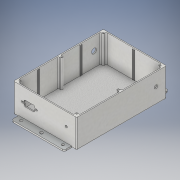
# Autodesk Inventor part: Main Enclosure Base
Saved by Autodesk Inventor 2019 (Build 230136000, 136)
## iProperties
Created: 2020-02-20
Part Number: Main Enclosure Base
Material: Generic
Document SubType Name: Modeling
Designer: gfb14170
Density: 1 g/cm^3
Appearance: Paint
Author: gfb14170
Autodesk Inventor part; units mm, degrees
ref_plane "YZ Plane" through (0, 0, 0) normal (1, 0, 0) x (0, 1, 0)
ref_plane "XZ Plane" through (0, 0, 0) normal (0, 1, 0) x (-1, 0, 0)
ref_plane "XY Plane" through (0, 0, 0) normal (0, 0, 1) x (1, 0, 0)
sketch "Sketch1" plane through (0, 0, 0) normal (0, 1, 0) x (-1, 0, 0)
  line L0 (60.4, 85.9) -> (-60.4, 85.9)
  line L1 (-60.4, 85.9) -> (-60.4, -85.9)
  line L2 (-60.4, -85.9) -> (60.4, -85.9)
  line L3 (60.4, -85.9) -> (60.4, 85.9)
  point P0 (0, 0)
  dimension "d0" = 85.9
  dimension "d1" = 85.9
  dimension "d2" = 60.4
  dimension "d3" = 60.4
  constraints: 8 end point, 2 parallel, 1 horizontal, 1 perpendicular
  measures "d0" distance from line of point (0, 0) L2
  measures "d1" distance from line of L0 point (0, 0)
  measures "d2" distance from line of point (0, 0) L3
  measures "d3" distance from line of L1 point (0, 0)
extrude "Extrusion1" add sketch "Sketch1" along normal blind 55.05
fillet "Fillet1" radius 2 6 edges at (60.4, 27.525, 85.9) (-60.4, 27.525, 85.9) (60.4, 27.525, -85.9) (-60.4, 27.525, -85.9) (60.4, 0, 0) (-60.4, 0, 0)
sketch "Sketch2" plane through (0, 55.05, 0) normal (0, 1, 0) x (1, 0, 0)
  line L0 (-58.4, -83.9) -> (58.4, -83.9)
  line L1 (58.4, -83.9) -> (58.4, 83.9)
  line L2 (58.4, 83.9) -> (-58.4, 83.9)
  line L3 (-58.4, 83.9) -> (-58.4, -83.9)
  line L4 (-60.4, 83.9) -> (-60.4, -83.9) projected
  line L5 (-58.4, -85.9) -> (58.4, -85.9) projected
  line L6 (60.4, -83.9) -> (60.4, 83.9) projected
  line L7 (58.4, 85.9) -> (-58.4, 85.9) projected
  point P0 (0, 0)
  dimension "d7" = 2
  dimension "d8" = 2
  dimension "d9" = 2
  dimension "d10" = 2
  constraints: 8 end point, 2 parallel, 1 horizontal, 1 perpendicular
  measures "d7" distance between parallel lines of L4 L3
  measures "d8" distance between parallel lines of L5 L0
  measures "d9" distance between parallel lines of L6 L1
  measures "d10" distance between parallel lines of L7 L2
extrude "Extrusion2" cut sketch "Sketch2" against normal blind 53.05
sketch "Sketch3" plane through (0, 0, 0) normal (0, -1, 0) x (1, 0, 0)
  line L0 (-58.4, -85.9) -> (-58.4, 85.9) projected
  line L1 (58.4, -85.9) -> (-58.4, -85.9) projected
  line L2 (58.4, 85.9) -> (58.4, -85.9) projected
  line L3 (-58.4, 85.9) -> (58.4, 85.9) projected
  line L4 (-58.4, 85.9) -> (58.4, 85.9) projected
  line L5 (50.4, 85.9) -> (50.4, 99.9)
  line L6 (50.4, 99.9) -> (-50.4, 99.9)
  line L7 (-50.4, 99.9) -> (-50.4, 85.9)
  line L8 (-60.4, 83.9) -> (-60.4, -83.9) projected
  line L9 (60.4, -83.9) -> (60.4, 83.9) projected
  line L10 (-134.6994, 0) -> (135.5184, 0) construction
  line L11 (50.4, -85.9) -> (50.4, -99.9)
  line L12 (50.4, -99.9) -> (-50.4, -99.9)
  line L13 (-50.4, -99.9) -> (-50.4, -85.9)
  line L14 (50.4, 85.9) -> (-50.4, 85.9)
  line L15 (-50.4, -85.9) -> (50.4, -85.9)
  point P0 (0, 0)
  dimension "d13" = 10
  dimension "d14" = 10
  dimension "d15" = 14
  dimension "d16" = 0
  constraints: 18 end point, 4 symmetric about line, 2 parallel, 1 collinear, 1 horizontal, 1 point on line
  measures "d13" distance between parallel lines of L8 L7
  measures "d14" distance between parallel lines of L5 L9
  measures "d15" distance between parallel lines of L3 L6
  measures "d16" distance from line of point (0, 0) L10
extrude "Extrusion3" add sketch "Sketch3" against normal blind 3 contours L1 L11 L12 L13 | L7 L6 L5 L3
fillet "Fillet2" radius 4 4 edges at (-50.4, 1.5, -99.9) (50.4, 1.5, -99.9) (50.4, 1.5, 99.9) (-50.4, 1.5, 99.9)
fillet "Fillet3" radius 2 8 edges at (-59.8142, 0.5858, 85.3142) (-54.4, 0, 85.9) (59.8142, 0.5858, 85.3142) (54.4, 0, 85.9) (59.8142, 0.5858, -85.3142) (54.4, 0, -85.9) (-59.8142, 0.5858, -85.3142) (-54.4, 0, -85.9)
sketch "Sketch4" plane through (0, 2, 0) normal (0, 1, 0) x (1, 0, 0)
  circle A0 centre (-54.9, 80.4) radius 1.25
  line L0 (58.4, 85.9) -> (-58.4, 85.9) projected
  line L1 (-60.4, 83.9) -> (-60.4, -83.9) projected
  circle A1 centre (54.1, 80.4) radius 1.25
  circle A2 centre (-54.9, -79.6) radius 1.25
  circle A3 centre (54.1, -79.6) radius 1.25
  circle A4 centre (-54.9, 80.4) radius 2.25
  circle A5 centre (-54.9, -79.6) radius 2.25
  circle A6 centre (54.1, 80.4) radius 2.25
  circle A7 centre (54.1, -79.6) radius 2.25
  line L2 (-58.4, 83.9) -> (-60.4, 83.9) projected
  line L3 (-58.4, 83.9) -> (-58.4, 75.9)
  line L4 (-58.4, 83.9) -> (-58.4, -83.9) projected
  line L5 (-58.4, 85.9) -> (-58.4, 83.9) projected
  line L6 (-58.4, 83.9) -> (-50.4, 83.9)
  line L7 (-58.4, 83.9) -> (58.4, 83.9) projected
  arc A8 (-55.4407, 78.2159) -> (-58.4, 75.9) centre (-56.0141, 75.9) ccw
  arc A9 (-50.4, 83.9) -> (-52.7159, 80.9407) centre (-50.4, 81.5141) ccw
  line L8 (58.4, 83.9) -> (58.4, -83.9) projected
  line L9 (58.4, 83.9) -> (50.4, 83.9)
  line L10 (58.4, 83.9) -> (58.4, 75.9)
  line L11 (58.4, -83.9) -> (58.4, 83.9) projected
  arc A10 (52.0522, 81.3323) -> (50.4, 83.9) centre (50.4, 82.0846) ccw
  arc A11 (58.4, 75.9) -> (54.9071, 78.2997) centre (55.8292, 75.9) ccw
  line L12 (58.4, -83.9) -> (-58.4, -83.9) projected
  line L13 (-58.4, -83.9) -> (-58.4, -75.9)
  line L14 (-58.4, -83.9) -> (-58.4, 83.9) projected
  line L15 (-58.4, -83.9) -> (-50.4, -83.9)
  arc A12 (-52.7997, -80.4071) -> (-50.4, -83.9) centre (-50.4, -81.3292) ccw
  arc A13 (-58.4, -75.9) -> (-55.8323, -77.5522) centre (-56.5846, -75.9) ccw
  line L16 (58.4, -83.9) -> (50.4, -83.9)
  line L17 (58.4, -83.9) -> (58.4, -75.9)
  arc A14 (55.2614, -77.6729) -> (58.4, -75.9) centre (56.33, -75.9) ccw
  arc A15 (50.4, -83.9) -> (52.1729, -80.7614) centre (50.4, -81.83) ccw
  circle A16 centre (54.5, 0) radius 1.25
  circle A17 centre (-54.5, 0) radius 1.25
  circle A18 centre (-54.5, 0) radius 2.25
  circle A19 centre (54.5, 0) radius 2.25
  line L18 (54.5, -2.25) -> (58.4, -2.25)
  line L19 (54.5, 2.25) -> (58.4, 2.25)
  line L20 (-54.5, -2.25) -> (-58.4, -2.25)
  line L21 (-54.5, 2.25) -> (-58.4, 2.25)
  line L22 (-58.4, -83.9) -> (-58.4, 83.9) projected
  line L23 (-58.4, 83.9) -> (58.4, 83.9) projected
  line L24 (58.4, 83.9) -> (58.4, -83.9) projected
  line L25 (58.4, -83.9) -> (-58.4, -83.9) projected
  point P0 (0, 0)
  dimension "d21" = 2.5
  dimension "d23" = 5.5
  dimension "d24" = 5.5
  dimension "d27" = 109
  dimension "d30" = 160
  dimension "d33" = 4.5
  dimension "d36" = 160
  dimension "d39" = 109
  dimension "d42" = 8
  dimension "d43" = 8
  dimension "d44" = 8
  dimension "d45" = 8
  dimension "d46" = 8
  dimension "d47" = 8
  dimension "d48" = 8
  dimension "d49" = 8
  dimension "d52" = 2.5
  dimension "d53" = 2.5
  dimension "d54" = 3.9
  dimension "d56" = 3.9
  dimension "d57" = 0
  dimension "d58" = 0
  dimension "d59" = 4.5
  dimension "d60" = 4.5
  constraints: 28 point on circle, 24 end point, 20 centre point, 20 tangent, 12 point on line, 3 coincident, 3 horizontal, 3 perpendicular, 2 vertical, 12 other
  measures "d21" diameter of A0
  measures "d23" distance from line of L0 A0.centre
  measures "d24" distance from line of L1 A0.centre
  measures "d27" distance of A0.centre A1.centre
  measures "d30" distance of A0.centre A2.centre
  measures "d33" diameter of A4
  measures "d36" distance of A4.centre A5.centre
  measures "d39" distance of A4.centre A6.centre
  measures "d42" distance of L2.start L3.end
  measures "d43" distance of L2.start L6.end
  measures "d44" distance of L7.end L9.end
  measures "d45" distance of L7.end L10.end
  measures "d46" distance of L4.end L13.end
  measures "d47" distance of L4.end L15.end
  measures "d48" distance of L8.end L16.end
  measures "d49" distance of L8.end L17.end
  measures "d52" diameter of A16
  measures "d53" diameter of A17
  measures "d54" distance from line of A16.centre L8
  measures "d56" distance from line of A17.centre L14
  measures "d57" vertical distance of A16.centre point (0, 0)
  measures "d58" vertical distance of point (0, 0) A17.centre
  measures "d59" diameter of A18
  measures "d60" diameter of A19
extrude "Extrusion4" add sketch "Sketch4" along normal up to surface (53.05 mm away) contours A4 | A4 A8 L3 L6 A9 | L7 L8 A11 A6 A10 | L21 A18 L20 L4 | A6 | A18 | A13 A5 A12 L12 L4 | L8 L18 A19 L19 | A5 | A19 | L8 L12 A15 A7 A14 | A7
fillet "Fillet4" radius 2 4 edges at (58.4, 28.525, -2.25) (58.4, 28.525, 2.25) (-58.4, 28.525, -2.25) (-58.4, 28.525, 2.25)
sketch "Sketch5" plane through (50.4, 55.05, 83.9) normal (0, 0, -1) x (-1, 0, 0)
  line L0 (0, -53.05) -> (100.8, -53.05) projected
  line L1 (48.5, -53.05) -> (49.5, -53.05)
  line L2 (49.5, -53.05) -> (49.5, -2)
  line L3 (49.5, -2) -> (48.5, -2)
  line L4 (48.5, -2) -> (48.5, -53.05)
  line L5 (-8, 0) -> (-8, -53.05) projected
  line L6 (0, 0) -> (100.8, 0) projected
  line L7 (52.5, -53.05) -> (52.5, -2)
  line L8 (51.5, -2) -> (51.5, -53.05)
  line L9 (52.5, -2) -> (51.5, -2)
  line L10 (51.5, -53.05) -> (52.5, -53.05)
  point P0 (50.4, -55.05)
  dimension "d75" = 56.5
  dimension "d76" = 1
  dimension "d77" = 2
  dimension "d80" = 3
  constraints: 16 end point, 2 horizontal, 2 parallel, 2 perpendicular, 1 point on line, 7 other
  measures "d75" distance between parallel lines of L5 L4
  measures "d76" distance between parallel lines of L2 L4
  measures "d77" distance between parallel lines of L6 L3
  measures "d80" distance of L1.end L7.start
sketch "Sketch6" plane through (0, 3, 0) normal (0, 1, 0) x (1, 0, 0)
  circle A0 centre (40.4, 92.9) radius 2.5
  line L0 (50.4, 85.9) -> (50.4, 95.9) projected
  line L1 (46.4, 99.9) -> (-46.4, 99.9) projected
  circle A1 centre (-39.6, 92.9) radius 2.5
  circle A2 centre (40.4, -92.1) radius 2.5
  circle A3 centre (-39.6, -92.1) radius 2.5
  circle A4 centre (0, 92.9) radius 3
  circle A5 centre (0, -92.9) radius 3
  line L2 (-50.4, -85.9) -> (50.4, -85.9) projected
  line L3 (0, 139.86) -> (0, -139.86) projected
  line L4 (50.4, 85.9) -> (-50.4, 85.9) projected
  point P0 (0, 0)
  dimension "d62" = 5
  dimension "d63" = 10
  dimension "d64" = 7
  dimension "d67" = 80
  dimension "d70" = 185
  dimension "d109" = 6
  dimension "d110" = 6
  dimension "d111" = 7
  dimension "d112" = 0
  dimension "d113" = 7
  dimension "d114" = 0
  constraints: 6 centre point, 1 horizontal, 1 vertical, 6 other
  measures "d62" diameter of A0
  measures "d63" distance from line of L0 A0.centre
  measures "d64" distance from line of L1 A0.centre
  measures "d67" distance of A0.centre A1.centre
  measures "d70" distance of A0.centre A2.centre
  measures "d109" diameter of A4
  measures "d110" diameter of A5
  measures "d111" distance from line of L2 A5.centre
  measures "d112" distance from line of L3 A5.centre
  measures "d113" distance from line of L4 A4.centre
  measures "d114" distance from line of L3 A4.centre
extrude "Extrusion5" cut sketch "Sketch6" against normal blind 3
extrude "Extrusion6" add sketch "Sketch5" along normal blind 1
sketch "Sketch7" plane through (58.4, 2, -75.9) normal (-1, 0, 0) x (0, 0, 1)
  line L0 (0, 0) -> (71.65, 0) projected
  line L1 (33.5, 0) -> (34.5, 0)
  line L2 (34.5, 0) -> (34.5, 51.05)
  line L3 (34.5, 51.05) -> (33.5, 51.05)
  line L4 (33.5, 51.05) -> (33.5, 0)
  line L5 (-8, 53.05) -> (-8, 0) projected
  line L6 (0, 53.05) -> (71.65, 53.05) projected
  line L7 (37.5, 0) -> (37.5, 51.05)
  line L8 (36.5, 51.05) -> (36.5, 0)
  line L9 (37.5, 51.05) -> (36.5, 51.05)
  line L10 (36.5, 0) -> (37.5, 0)
  line L11 (-8, 0) -> (159.8, 0) projected
  line L12 (118.3, 0) -> (117.3, 0)
  line L13 (117.3, 0) -> (117.3, 51.05)
  line L14 (117.3, 51.05) -> (118.3, 51.05)
  line L15 (118.3, 51.05) -> (118.3, 0)
  line L16 (159.8, 53.05) -> (159.8, 0) projected
  line L17 (80.15, 53.05) -> (151.8, 53.05) projected
  line L18 (114.3, 0) -> (114.3, 51.05)
  line L19 (115.3, 51.05) -> (115.3, 0)
  line L20 (114.3, 51.05) -> (115.3, 51.05)
  line L21 (115.3, 0) -> (114.3, 0)
  point P0 (75.9, -2)
  dimension "d87" = 41.5
  dimension "d88" = 1
  dimension "d89" = 2
  dimension "d92" = 3
  dimension "d97" = 41.5
  dimension "d98" = 1
  dimension "d99" = 2
  dimension "d102" = 3
  constraints: 32 end point, 4 horizontal, 4 parallel, 2 perpendicular, 1 point on line, 18 other
  measures "d87" distance between parallel lines of L5 L4
  measures "d88" distance between parallel lines of L4 L2
  measures "d89" distance between parallel lines of L6 L3
  measures "d92" distance of L1.end L7.start
  measures "d97" distance between parallel lines of L16 L15
  measures "d98" distance between parallel lines of L15 L13
  measures "d99" distance between parallel lines of L17 L14
  measures "d102" distance of L12.end L18.start
extrude "Extrusion7" add sketch "Sketch7" along normal blind 1
mirror "Mirror1" about plane through (0, 0, 0) normal (1, 0, 0) of "Extrusion7"
mirror "Mirror2" about plane through (0, 0, 0) normal (0, 0, 1) of "Extrusion6"
sketch "Sketch9" plane through (-60.4, 55.05, -83.9) normal (-1, 0, 0) x (0, 0, 1)
  circle A0 centre (18, -25) radius 4.75
  line L0 (169.8, -53.05) -> (169.8, 0) projected
  line L1 (0, 0) -> (167.8, 0) projected
  line L2 (-2, 0) -> (-2, -53.05) projected
  point P0 (83.9, -55.05)
  dimension "d115" = 9.5
  dimension "d120" = 25
  dimension "d121" = 20
  constraints: 1 centre point
  measures "d115" diameter of A0
  measures "d120" distance from line of L1 A0.centre
  measures "d121" distance from line of L2 A0.centre
extrude "Extrusion8" cut sketch "Sketch9" against normal up to surface (2 mm away)
sketch "Sketch10" plane through (-58.4, 55.05, 85.9) normal (0, 0, 1) x (1, 0, 0)
  line L0 (20, -20.55) -> (36.5, -20.55)
  line L1 (38, -22.05) -> (38, -30.05)
  line L2 (36.5, -31.55) -> (19.5, -31.55)
  line L3 (18, -30.05) -> (18, -22.55)
  line L4 (104.8, -55.05) -> (12, -55.05) projected
  line L5 (-2, 0) -> (-2, -53.05) projected
  line L6 (11.4715, -26.05) -> (47.4715, -26.05) construction
  arc A0 (13.9, -24.55) -> (13.9, -27.55) centre (13.9, -26.05) ccw
  arc A1 (42.1, -27.55) -> (42.1, -24.55) centre (42.1, -26.05) ccw
  line L7 (28, -13.0894) -> (28, -41.0894) construction
  arc A2 (20, -20.55) -> (18, -22.55) centre (20, -22.55) ccw
  arc A3 (38, -22.05) -> (36.5, -20.55) centre (36.5, -22.05) ccw
  arc A4 (36.5, -31.55) -> (38, -30.05) centre (36.5, -30.05) ccw
  arc A5 (18, -30.05) -> (19.5, -31.55) centre (19.5, -30.05) ccw
  line L8 (13.9, -24.55) -> (18, -24.55)
  line L9 (13.9, -27.55) -> (18, -27.55)
  line L10 (42.1, -27.55) -> (38, -27.55)
  line L11 (42.1, -24.55) -> (38, -24.55)
  point P0 (58.4, -55.05)
  dimension "d122" = 11
  dimension "d123" = 20
  dimension "d124" = 23.5
  dimension "d125" = 20
  dimension "d126" = 5.5
  dimension "d127" = 3
  dimension "d128" = 3
  dimension "d129" = 10
  dimension "d130" = 14.1
  dimension "d131" = 14.1
  dimension "d132" = 2
  dimension "d133" = 1.5
  constraints: 20 end point, 12 point on circle, 10 point on line, 10 tangent, 6 centre point, 3 perpendicular, 2 equal radius, 2 horizontal, 2 parallel, 1 vertical
  measures "d122" distance between parallel lines of L0 L2
  measures "d123" distance between parallel lines of L1 L3
  measures "d124" distance between parallel lines of L4 L2
  measures "d125" distance between parallel lines of L5 L3
  measures "d126" distance between parallel lines of L0 L6
  measures "d127" diameter of A0
  measures "d128" diameter of A1
  measures "d129" distance between parallel lines of L3 L7
  measures "d130" distance from line of A0.centre L7
  measures "d131" distance from line of L7 A1.centre
  measures "d132" radius of A2
  measures "d133" radius of A3
extrude "Extrusion9" cut sketch "Sketch10" against normal up to surface (2 mm away)
sketch "Sketch11" plane through (-58.4, 55.05, 85.9) normal (0, 0, 1) x (1, 0, 0)
  circle A0 centre (98.8, -25) radius 2.1
  line L0 (0, 0) -> (116.8, 0) projected
  line L1 (118.8, -53.05) -> (118.8, 0) projected
  point P0 (58.4, -55.05)
  dimension "d136" = 4.2
  dimension "d137" = 25
  dimension "d138" = 20
  constraints: 1 centre point
  measures "d136" diameter of A0
  measures "d137" distance from line of L0 A0.centre
  measures "d138" distance from line of L1 A0.centre
extrude "Extrusion10" cut sketch "Sketch11" against normal up to surface (2 mm away)
sketch "Sketch12" plane through (60.4, 55.05, 83.9) normal (1, 0, 0) x (0, 0, -1)
  circle A0 centre (149.8, -25) radius 4.75 projected
  circle A1 centre (149.8, -25) radius 3.25
  point P0 (83.9, -55.05)
  dimension "d141" = 3.25
  constraints: 1 centre point, 1 coincident
  measures "d141" radius of A1
extrude "Extrusion11" cut sketch "Sketch12" against normal blind 10 contours A1
equation "\"d1\" = d0"
equation "\"d3\" = d2"
equation "\"d7\" = d8"
equation "\"d9\" = d8"
equation "\"d10\" = d8"
equation "\"d126\" = 0.5 * d122"
equation "\"d129\" = 0.5 * d123"
equation "\"d131\" = d130"
body "Solid1"
